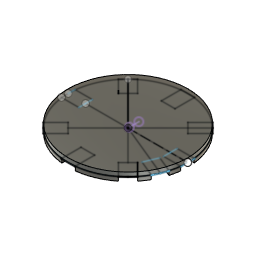
Universalen Teller v1 (Autodesk Fusion 360 design; units mm, degrees)
Autodesk Fusion 360 part; units mm, degrees
sketch "Skizze1" plane through (0, 0, 0) normal (0, 0, 1) x (1, 0, 0)
  circle A0 centre (0, 0) radius 110
  line L0 (-12.5, 110) -> (12.5, 110)
  line L1 (12.5, 110) -> (12.5, 74)
  line L2 (12.5, 74) -> (-12.5, 74)
  line L3 (-12.5, 74) -> (-12.5, 110)
  line L4 (0, 0) -> (77.7817, 77.7817)
  line L5 (0, 0) -> (110, 0) construction
  line L6 (0, 0) -> (-77.7817, 77.7817)
  line L7 (0, 0) -> (110, 0) construction
  line L8 (77.7817, 77.7817) -> (68.9429, 86.6206)
  line L9 (77.7817, 77.7817) -> (86.6206, 68.9429)
  line L10 (86.6206, 68.9429) -> (63.9932, 46.3155)
  line L11 (68.9429, 86.6206) -> (46.3155, 63.9932)
  line L12 (46.3155, 63.9932) -> (63.9932, 46.3155)
  line L13 (0, 2.5) -> (0, 20)
  line L14 (-86.6206, 68.9429) -> (-63.9932, 46.3155)
  line L15 (-46.3155, 63.9932) -> (-63.9932, 46.3155)
  line L16 (-68.9429, 86.6206) -> (-46.3155, 63.9932)
  line L17 (-77.7817, 77.7817) -> (-68.9429, 86.6206)
  line L18 (-77.7817, 77.7817) -> (-86.6206, 68.9429)
  line L19 (110, 0) -> (78, 0)
  line L20 (78, 0) -> (78, 12.5)
  line L21 (78, 12.5) -> (110, 12.5)
  line L22 (110, 12.5) -> (110, 0)
  line L23 (-78, 0) -> (-78, 12.5)
  line L24 (-78, 12.5) -> (-110, 12.5)
  line L25 (-110, 12.5) -> (-110, 0)
  line L26 (-78, -12.5) -> (-110, -12.5)
  line L27 (-78, 0) -> (-78, -12.5)
  line L28 (-86.6206, -68.9429) -> (-63.9932, -46.3155)
  line L29 (-77.7817, -77.7817) -> (-86.6206, -68.9429)
  line L30 (-77.7817, -77.7817) -> (-68.9429, -86.6206)
  line L31 (-68.9429, -86.6206) -> (-46.3155, -63.9932)
  line L32 (-46.3155, -63.9932) -> (-63.9932, -46.3155)
  line L33 (12.5, -74) -> (-12.5, -74)
  line L34 (12.5, -110) -> (12.5, -74)
  line L35 (-12.5, -74) -> (-12.5, -110)
  line L36 (-12.5, -110) -> (12.5, -110)
  line L37 (77.7817, -77.7817) -> (68.9429, -86.6206)
  line L38 (77.7817, -77.7817) -> (86.6206, -68.9429)
  line L39 (86.6206, -68.9429) -> (63.9932, -46.3155)
  line L40 (46.3155, -63.9932) -> (63.9932, -46.3155)
  line L41 (68.9429, -86.6206) -> (46.3155, -63.9932)
  line L42 (78, 0) -> (78, -12.5)
  line L43 (78, -12.5) -> (110, -12.5)
  line L44 (110, -12.5) -> (110, 0)
  line L45 (0, 0) -> (-55.1543, -55.1543)
  line L46 (0, 0) -> (55.1543, -55.1543)
  line L47 (0, 0) -> (-78, 0)
  line L48 (0, 0) -> (78, 0)
  line L49 (0, 0) -> (101.6267, -42.0952)
  line L50 (0, 0) -> (110, 0) construction
  line L51 (101.6267, -42.0952) -> (96.8432, -53.6437)
  line L52 (101.6267, -42.0952) -> (106.4103, -30.5467)
  line L53 (96.8432, -53.6437) -> (67.2791, -41.3978)
  line L54 (106.4103, -30.5467) -> (76.8461, -18.3008)
  line L55 (67.2791, -41.3978) -> (76.8461, -18.3008)
  dimension "d1" = 25
  dimension "d2" = 36
  dimension "d3" = 12.5
  dimension "d4" = 110
  dimension "d5" = 45
  dimension "d6" = 135
  dimension "d7" = 12.5
  dimension "d8" = 12.5
  dimension "d9" = 32
  dimension "d10" = 32
  dimension "d11" = 32
  dimension "d12" = 12.5
  dimension "d13" = 22.5
  dimension "d14" = 12.5
  dimension "d15" = 12.5
  dimension "d16" = 32
  dimension "d17" = 32
  constraint coincident A0.centre L4.start
  constraint horizontal L0
  constraint vertical L1
  constraint horizontal L2
  constraint vertical L3
  constraint horizontal L5
  constraint horizontal L7
  constraint tangent A0 L8
  constraint perpendicular L4 L8
  constraint tangent A0 L9
  constraint perpendicular L4 L9
  constraint perpendicular L8 L10
  constraint perpendicular L8 L11
  constraint symmetric L4.end L13 L6.end
  constraint symmetric L8.end L13 L16.start
  constraint symmetric L9.end L13 L14.start
  constraint symmetric L10.end L13 L14.end
  constraint symmetric L11.end L13 L15.start
  constraint horizontal L19
  constraint vertical L20
  constraint horizontal L21
  constraint vertical L22
  constraint symmetric L5.end L13 L25.end
  constraint symmetric L13 L19.end L23.start
  constraint symmetric L13 L20.end L23.end
  constraint symmetric L13 L21.end L24.end
  constraint symmetric L0.start L7 L35.end
  constraint symmetric L0.end L7 L34.start
  constraint symmetric L1.end L7 L33.start
  constraint symmetric L2.end L7 L33.end
  constraint symmetric L4.end L7 L37.start
  constraint symmetric L5.end L7 L19.start
  constraint symmetric L7 L8.end L37.end
  constraint symmetric L7 L9.end L38.end
  constraint symmetric L7 L10.end L39.end
  constraint symmetric L7 L11.end L40.start
  constraint symmetric L7 L14.start L28.start
  constraint symmetric L7 L14.end L28.end
  constraint symmetric L7 L15.start L31.end
  constraint symmetric L7 L16.start L30.end
  constraint symmetric L7 L6.end L29.start
  constraint symmetric L7 L19.end L20.start
  constraint symmetric L7 L20.end L42.end
  constraint symmetric L7 L21.end L43.end
  constraint symmetric L7 L24.end L26.end
  constraint symmetric L7 L23.start L27.start
  constraint symmetric L7 L23.end L26.start
  constraint midpoint L32 L45.end
  constraint midpoint L40 L46.end
  constraint horizontal L50
  constraint perpendicular L49 L51
  constraint perpendicular L49 L52
  constraint perpendicular L51 L53
  constraint perpendicular L52 L54
  measures "d1" distance of L0.start L0.end
  measures "d2" distance of L0.start L2.end
  measures "d3" distance of A0.centre L3
  measures "d4" distance of A0.centre L0
  measures "d5" angle of L4 L5
  measures "d6" angle of L6 L7
  measures "d7" distance of L4.end L8.end
  measures "d8" distance of L4.end L9.end
  measures "d9" distance of L9.end L10.end
  measures "d10" distance of L8.end L11.end
  measures "d11" distance of L5.end L19.end
  measures "d12" distance of L5.end L21.end
  measures "d13" angle of L49 L50
  measures "d14" distance of L49.end L51.end
  measures "d15" distance of L49.end L52.end
  measures "d16" distance of L51.end L53.end
  measures "d17" distance of L52.end L54.end
extrude "Extrusion1" add sketch "Skizze1" along normal blind 7.5 contours A0 L19 L20 L21 | A0 L19 L42 L43 | A0 L4 L10 L12 L20 L21 L48 | A0 L42 L43 L48 L49 L54 L55 | A0 L4 L10 L12 | A0 L49 L54 L55 | A0 L1 L2 L3 L4 L6 L11 L12 L15 L16 | A0 L6 L14 L15 L23 L24 L47 | A0 L31 L32 L33 L34 L35 L40 L41 L45 L46 | A0 L39 L40 L46 L49 L53 L55 | A0 L26 L27 L28 L32 L45 L47 | A0 L4 L11 L12 | A0 L49 L53 L55 | A0 L6 L14 L15 | A0 L6 L15 L16 | A0 L28 L31 L32 | A0 L39 L40 L41 | A0 L23 L24 L26 L27 | A0 L1 L2 L3 | A0 L33 L34 L35 makes body 1
extrude "Extrusion2" add sketch "Skizze1" against normal blind 7.5 separate body contours A0 L4 L10 L12 L20 L21 L48 | A0 L42 L43 L48 L49 L54 L55 | A0 L1 L2 L3 L4 L6 L11 L12 L15 L16 | A0 L6 L14 L15 L23 L24 L47 | A0 L31 L32 L33 L34 L35 L40 L41 L45 L46 | A0 L39 L40 L46 L49 L53 L55 | A0 L26 L27 L28 L32 L45 L47 makes body 2
